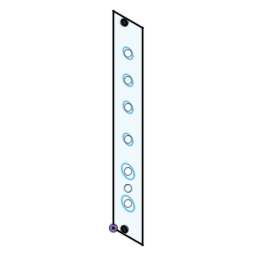
FU-CADETII-RGBNCODER v6 (Autodesk Fusion 360 design; units mm, degrees)
Autodesk Fusion 360 part; units mm, degrees
sketch "Sketch1" plane through (0, 0, 0) normal (0, 1, 0) x (1, 0, 0)
  line L0 (0, 0) -> (20, 0)
  line L1 (20, 0) -> (20, -128.5)
  line L2 (20, -128.5) -> (0, -128.5)
  line L3 (0, -128.5) -> (0, 0)
  circle A0 centre (10, -108.5) radius 3.16
  circle A1 centre (10, -92.5) radius 3.16
  circle A2 centre (7.5, -125.5) radius 1.6
  circle A3 centre (10, -57.5) radius 3.16
  circle A4 centre (10, -38.5) radius 4.25
  circle A5 centre (10, -76.5) radius 3.16
  circle A6 centre (10, -28.5) radius 1.75
  circle A7 centre (7.5, -3) radius 1.6
  circle A8 centre (10, -19.5) radius 4.25
  dimension "d1" = 20
  dimension "d2" = 128.5
  dimension "d3" = 6.32
  dimension "d5" = 6.32
  dimension "d6" = 36
  dimension "d7" = 3.2
  dimension "d8" = 7.5
  dimension "d9" = 6.32
  dimension "d10" = 71
  dimension "d11" = 8.5
  dimension "d12" = 6.32
  dimension "d13" = 3.5
  dimension "d14" = 90
  dimension "d15" = 52
  dimension "d16" = 100
  dimension "d17" = 3
  dimension "d18" = 3.2
  dimension "d19" = 3
  dimension "d20" = 7.5
  dimension "d21" = 8.5
  dimension "d22" = 109
  constraint horizontal L0
  constraint vertical L1
  constraint horizontal L2
  constraint vertical L3
  constraint coincident L0.start L3.end
  measures "d1" distance of L1.end L2.end
  measures "d2" distance of L0.end L1.end
  measures "d3" diameter of A0
  measures "d5" diameter of A1
  measures "d6" distance of L2 A1.centre
  measures "d7" diameter of A2
  measures "d8" distance of L3 A2.centre
  measures "d9" diameter of A3
  measures "d10" distance of L2 A3.centre
  measures "d11" diameter of A4
  measures "d12" diameter of A5
  measures "d13" diameter of A6
  measures "d14" distance of L2 A4.centre
  measures "d15" distance of L2 A5.centre
  measures "d16" distance of L2 A6.centre
  measures "d17" distance of L2 A2.centre
  measures "d18" diameter of A7
  measures "d19" distance of L0 A7.centre
  measures "d20" distance of L3 A7.centre
  measures "d21" diameter of A8
  measures "d22" distance of L2 A8.centre
extrude "Extrude1" add sketch "Sketch1" along normal blind 2
hidden bodies 1
equation "d5 = d3"
equation "d6 = 27 mm + 9 mm"
equation "d9 = d3"
equation "d10 = 62 mm + 9 mm"
equation "d12 = d3"
equation "d14 = 81 mm + 9 mm"
equation "d15 = 43 mm + 9 mm"
